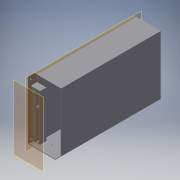
# Autodesk Inventor part: PSU
Saved by Autodesk Inventor 2018 (Build 220112000, 112)
## iProperties
Created: 2018-05-17
Part Number: PSU
Material: Generic
Document SubType Name: Modeling
Designer: Jasper
Density: 1 g/cm^3
Appearance: Default
Author: Jasper
Autodesk Inventor part; units mm, degrees
ref_plane "YZ Plane" through (0, 0, 0) normal (1, 0, 0) x (0, 1, 0)
ref_plane "XZ Plane" through (0, 0, 0) normal (0, 1, 0) x (-1, 0, 0)
ref_plane "XY Plane" through (0, 0, 0) normal (0, 0, 1) x (1, 0, 0)
sketch "Sketch1" plane through (0, 0, 0) normal (0, 1, 0) x (-1, 0, 0)
  line L0 (-25.425, 54.65) -> (25.425, 54.65)
  line L1 (25.425, 54.65) -> (25.425, -54.65)
  line L2 (25.425, -54.65) -> (-25.425, -54.65)
  line L3 (-25.425, -54.65) -> (-25.425, 54.65)
  line L4 (-25.425, 54.65) -> (25.425, -54.65) construction
  line L5 (25.425, 54.65) -> (-25.425, -54.65) construction
  point P0 (0, 0)
  dimension "d0" = 109.3
  dimension "d1" = 50.85
  constraints: 12 end point, 2 midpoint, 2 parallel, 1 horizontal, 1 perpendicular
  measures "d0" distance of L0.end L1.end
  measures "d1" distance of L1.end L2.end
extrude "Extrusion1" add sketch "Sketch1" along normal blind 185
shell "Shell1" thickness 1 removed faces 1 at (8.475, 0, 18.2167)
sketch "Sketch2" plane through (0, 0, 0) normal (0, -1, 0) x (1, 0, 0)
  line L0 (-24.425, -53.65) -> (-24.425, 53.65) projected
  line L1 (-24.425, 53.65) -> (24.425, 53.65) projected
  line L2 (24.425, 53.65) -> (24.425, -53.65) projected
  line L3 (24.425, -53.65) -> (-24.425, -53.65) projected
  line L4 (25.425, 54.65) -> (-25.425, 54.65) projected
  line L5 (-25.425, 54.65) -> (-25.425, -54.65) projected
  line L6 (-25.425, -54.65) -> (25.425, -54.65) projected
  line L7 (25.425, -54.65) -> (25.425, 54.65) projected
  line L8 (-24.425, 53.65) -> (-24.425, 54.65)
  line L9 (25.425, 54.65) -> (-25.425, 54.65) projected
  line L10 (24.425, 53.65) -> (24.425, -53.65) projected
  line L11 (24.425, -53.65) -> (25.425, -53.65)
  line L12 (25.425, -54.65) -> (25.425, 54.65) projected
  point P0 (0, 0)
  constraints: 4 end point, 2 perpendicular, 2 point on line
extrude "Extrusion2" add sketch "Sketch2" along normal blind 10.9 contours L3 L11 L7 L6 L5 L4 L8 L0
sketch "Sketch3" plane through (25.425, 185, -54.65) normal (0, 0, -1) x (-1, 0, 0)
  line L0 (0, -176.75) -> (50.85, -176.75) construction
  line L1 (50.85, 0) -> (50.85, -195.9) construction
  circle A0 centre (25.425, -176.75) radius 1.5
  line L2 (50.85, -195.9) -> (0, -195.9) projected
  line L3 (0, 0) -> (0, -195.9) projected
  line L4 (25.425, -176.75) -> (25.425, -38.45) construction
  circle A1 centre (25.425, -38.45) radius 1.5
  line L5 (25.425, -38.45) -> (39.825, -38.45) construction
  line L6 (39.825, -38.45) -> (39.825, -17.85) construction
  circle A2 centre (39.825, -17.85) radius 1.5
  point P0 (25.425, -185)
  dimension "d7" = 19.15
  dimension "d8" = 3
  dimension "d9" = 138.3
  dimension "d10" = 3
  dimension "d11" = 14.4
  dimension "d12" = 20.6
  dimension "d13" = 3
  constraints: 8 end point, 3 centre point, 2 coincident, 2 horizontal, 2 point on line, 1 midpoint, 1 perpendicular, 1 vertical
  measures "d7" distance between parallel lines of L2 L0
  measures "d8" diameter of A0
  measures "d9" distance of L4.start L4.end
  measures "d10" diameter of A1
  measures "d11" distance of L5.start L5.end
  measures "d12" distance of L5.end L6.end
  measures "d13" diameter of A2
extrude "Extrusion3" cut sketch "Sketch3" against normal up to surface (1 mm away)
sketch "Sketch4" plane through (-25.425, 185, -54.65) normal (-1, 0, 0) x (0, 0, 1)
  line L0 (0, -191.45) -> (109.3, -191.45) construction
  line L1 (109.3, 0) -> (109.3, -195.9) construction
  line L2 (109.3, -195.9) -> (0, -195.9) construction
  line L3 (0, 0) -> (0, -195.9) construction
  circle A0 centre (6.3, -191.45) radius 1.5
  circle A1 centre (102.3, -191.45) radius 1.5
  line L4 (0, -134.85) -> (109.3, -134.85) construction
  circle A2 centre (14.75, -134.85) radius 1.5
  circle A3 centre (99.8, -134.85) radius 1.5
  line L5 (0, -18.65) -> (109.3, -18.65) construction
  circle A4 centre (102.6, -18.65) radius 1.5
  line L6 (0, -8.85) -> (109.3, -8.85) construction
  circle A5 centre (14.6, -8.85) radius 1.5
  circle A6 centre (99.4, -8.85) radius 1.5
  point P0 (54.65, -185)
  dimension "d16" = 4.45
  dimension "d17" = 7
  dimension "d18" = 3
  dimension "d19" = 6.3
  dimension "d20" = 3
  dimension "d21" = 56.6
  dimension "d22" = 14.75
  dimension "d23" = 9.5
  dimension "d24" = 3
  dimension "d25" = 3
  dimension "d26" = 116.2
  dimension "d27" = 6.7
  dimension "d28" = 3
  dimension "d29" = 9.8
  dimension "d30" = 9.9
  dimension "d31" = 3
  dimension "d32" = 14.6
  dimension "d33" = 3
  constraints: 15 point on line, 8 end point, 7 centre point, 2 horizontal, 2 perpendicular
  measures "d16" distance between parallel lines of L2 L0
  measures "d17" distance from line of L1 A1.centre
  measures "d18" diameter of A1
  measures "d19" distance from line of L3 A0.centre
  measures "d20" diameter of A0
  measures "d21" distance between parallel lines of L0 L4
  measures "d22" distance from line of L3 A2.centre
  measures "d23" distance from line of L1 A3.centre
  measures "d24" diameter of A2
  measures "d25" diameter of A3
  measures "d26" distance between parallel lines of L4 L5
  measures "d27" distance from line of L1 A4.centre
  measures "d28" diameter of A4
  measures "d29" distance between parallel lines of L5 L6
  measures "d30" distance from line of L1 A6.centre
  measures "d31" diameter of A6
  measures "d32" distance from line of L3 A5.centre
  measures "d33" diameter of A5
extrude "Extrusion4" cut sketch "Sketch4" against normal up to surface (1 mm away)
ref_plane "Work Plane1" through (-19.425, 0, 53.65) normal (1, 0, 0) x (0, 0, -1)
sketch "Sketch5" plane through (-19.425, 0, 53.65) normal (1, 0, 0) x (0, 0, -1)
  line L0 (107.3, -10.9) -> (-1, -10.9) projected
  line L1 (97.3, -10.9) -> (97.3, 0)
  line L2 (107.3, 0) -> (107.3, -10.9) projected
  line L3 (11, -10.9) -> (11, 0)
  line L4 (-1, 0) -> (-1, -10.9) projected
  line L5 (11, -10.9) -> (97.3, -10.9)
  line L6 (11, 0) -> (-1, 0)
  line L7 (-1, 185) -> (-1, -10.9) projected
  line L8 (97.3, 0) -> (107.3, 0)
  line L9 (107.3, -10.9) -> (107.3, 184) projected
  line L10 (-1, 0) -> (11, 0)
  line L11 (0, 0) -> (0, 184) projected
  line L12 (0, 0) -> (0, 50)
  line L13 (0, 50) -> (107.3, 50)
  line L14 (107.3, 50) -> (107.3, 0)
  point P0 (53.65, 0)
  dimension "d36" = 10
  dimension "d37" = 12
  dimension "d38" = 50
  constraints: 18 end point, 5 perpendicular, 4 point on line, 2 collinear, 1 horizontal
  measures "d36" distance between parallel lines of L2 L1
  measures "d37" distance between parallel lines of L4 L3
  measures "d38" distance between parallel lines of L8 L13
extrude "Extrusion5" add sketch "Sketch5" along normal blind 1.5 contours L0 L3 L6 L11 L13 L9 L8 L1
sketch "Sketch6" plane through (-17.925, 0, 53.65) normal (1, 0, 0) x (0, 0, -1)
  line L0 (97.3, 0) -> (107.3, 0) projected
  line L1 (97.3, 0) -> (11, 0)
  line L2 (11, 0) -> (11, -11.9)
  line L3 (11, -11.9) -> (97.3, -11.9)
  line L4 (97.3, -11.9) -> (97.3, 0)
  line L5 (11, 0) -> (11, -10.9) projected
  line L6 (11, -10.9) -> (97.3, -10.9) projected
  point P0 (53.65, 0)
  dimension "d42" = 1
  constraints: 8 end point, 2 parallel, 1 collinear, 1 horizontal, 1 perpendicular
  measures "d42" distance between parallel lines of L3 L6
extrude "Extrusion6" add sketch "Sketch6" along normal blind 16
sketch "Sketch7" plane through (-17.925, -11.9, -43.65) normal (0, -1, 0) x (1, 0, 0)
  line L0 (13.5, 84.8) -> (8.5, 84.8)
  line L1 (8.5, 84.8) -> (8.5, 57.8)
  line L2 (8.5, 57.8) -> (13.5, 57.8)
  line L3 (13.5, 57.8) -> (13.5, 84.8)
  line L4 (0, 86.3) -> (16, 86.3) projected
  line L5 (16, 86.3) -> (16, 0) projected
  line L6 (0, 86.3) -> (0, 0) projected
  line L7 (13.5, 56.3) -> (8.5, 56.3)
  line L8 (8.5, 56.3) -> (8.5, 1.5)
  line L9 (8.5, 1.5) -> (13.5, 1.5)
  line L10 (13.5, 1.5) -> (13.5, 56.3)
  line L11 (0, 0) -> (16, 0) projected
  point P0 (17.925, 43.65)
  dimension "d45" = 1.5
  dimension "d46" = 2.5
  dimension "d47" = 27
  dimension "d48" = 8.5
  dimension "d49" = 1.5
  dimension "d50" = 1.5
  constraints: 16 end point, 4 parallel, 2 collinear, 2 horizontal, 2 perpendicular
  measures "d45" distance between parallel lines of L4 L0
  measures "d46" distance between parallel lines of L3 L5
  measures "d47" distance of L2.end L0.start
  measures "d48" distance between parallel lines of L6 L1
  measures "d49" distance between parallel lines of L2 L7
  measures "d50" distance between parallel lines of L11 L9
extrude "Extrusion7" cut sketch "Sketch7" against normal blind 16 contours L3 L2 L1 L0 | L10 L9 L8 L7
ref_plane "Work Plane2" through (0, -35.9, 0) normal (0, -1, 0) x (1, 0, 0)
ref_plane "Work Plane3" through (-25.425, 185, 0) normal (0, 0, 1) x (1, 0, 0)
body "Solid1"
